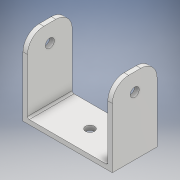
# Autodesk Inventor part: ShoulderPart2
Saved by Autodesk Inventor 2018 (Build 220112000, 112)
## iProperties
Created: 2018-02-09
Part Number: ShoulderPart2
Material: Plastique ABS
Document SubType Name: Modeling
Designer: Thomas
Density: 1.06 g/cm^3
Appearance: Lisse - Blanc
Author: Thomas
Autodesk Inventor part; units mm, degrees
ref_plane "YZ Plane" through (0, 0, 0) normal (1, 0, 0) x (0, 1, 0)
ref_plane "XZ Plane" through (0, 0, 0) normal (0, 1, 0) x (-1, 0, 0)
ref_plane "XY Plane" through (0, 0, 0) normal (0, 0, 1) x (1, 0, 0)
sketch "Esquisse1" plane through (0, 0, 0) normal (0, 0, 1) x (1, 0, 0)
  line L0 (0, 0) -> (98.8, 0)
  line L1 (98.8, 0) -> (98.8, 49.4)
  line L2 (98.8, 49.4) -> (0, 49.4)
  line L3 (0, 49.4) -> (0, 0)
  dimension "d0" = 98.8
  dimension "d1" = 49.4
  constraints: 8 end point, 2 parallel, 1 horizontal, 1 perpendicular
  measures "d0" distance of L1.end L2.end
  measures "d1" distance of L2.end L0.start
extrude "Extrusion1" add sketch "Esquisse1" along normal blind 5
sketch "Esquisse2" plane through (98.8, 0, 0) normal (1, 0, 0) x (0, 0, -1)
  line L0 (0, 49.4) -> (-5, 49.4) projected
  line L1 (-5, 49.4) -> (-66.3, 49.4)
  line L2 (-84.3, 31.4) -> (-84.3, 18)
  line L3 (-66.3, 0) -> (-5, 0)
  line L4 (-5, 0) -> (-5, 49.4)
  arc A0 (-66.3, 49.4) -> (-84.3, 31.4) centre (-66.3, 31.4) ccw
  arc A1 (-84.3, 18) -> (-66.3, 0) centre (-66.3, 18) ccw
  point P0 (0, 0)
  point P1 (-84.3, 49.4)
  dimension "d4" = 79.3
  dimension "d5" = 49.4
  dimension "d6" = 18
  dimension "d7" = 18
  constraints: 8 end point, 4 point on circle, 4 tangent, 2 centre point, 2 parallel, 2 point on line, 1 horizontal, 1 perpendicular
  measures "d4" distance of L0.end point (-84.3, 49.4)
  measures "d5" distance of L3.end L0.end
  measures "d6" radius of A0
  measures "d7" radius of A1
extrude "Extrusion2" add sketch "Esquisse2" against normal blind 5
sketch "Esquisse3" plane through (0, 0, 0) normal (-1, 0, 0) x (0, 0, 1)
  line L0 (66.3, 49.4) -> (5, 49.4) projected
  line L1 (5, 49.4) -> (66.3, 49.4)
  line L2 (84.3, 31.4) -> (84.3, 18)
  line L3 (66.3, 0) -> (5, 0)
  line L4 (5, 0) -> (5, 49.4)
  arc A0 (66.3, 0) -> (84.3, 18) centre (66.3, 18) ccw
  arc A1 (84.3, 31.4) -> (66.3, 49.4) centre (66.3, 31.4) ccw
  point P0 (0, 0)
  point P1 (84.3, 0)
  dimension "d13" = 79.3
  dimension "d14" = 49.4
  dimension "d15" = 18
  constraints: 8 end point, 4 point on circle, 4 tangent, 2 centre point, 2 parallel, 2 point on line, 1 equal radius, 1 horizontal, 1 perpendicular
  measures "d13" distance of point (84.3, 0) L3.end
  measures "d14" distance of L3.end L0.end
  measures "d15" radius of A0
extrude "Extrusion3" add sketch "Esquisse3" against normal blind 5
sketch "Esquisse4" plane through (0, 0, 0) normal (-1, 0, 0) x (0, 0, 1)
  circle A0 centre (64.8, 24.7) radius 5
  line L0 (84.3, 31.4) -> (84.3, 18) projected
  line L1 (0, 0) -> (66.3, 0) projected
  dimension "d18" = 10
  dimension "d19" = 19.5
  dimension "d20" = 24.7
  constraints: 1 centre point
  measures "d18" diameter of A0
  measures "d19" distance from line of L0 A0.centre
  measures "d20" distance from line of L1 A0.centre
extrude "Extrusion4" cut sketch "Esquisse4" against normal blind 5
sketch "Esquisse5" plane through (98.8, 0, 0) normal (1, 0, 0) x (0, 0, -1)
  circle A0 centre (-64.8, 24.7) radius 5
  line L0 (0, 49.4) -> (-66.3, 49.4) projected
  line L1 (-84.3, 31.4) -> (-84.3, 18) projected
  point P0 (0, 0)
  dimension "d23" = 10
  dimension "d24" = 24.7
  dimension "d25" = 19.5
  constraints: 1 centre point
  measures "d23" diameter of A0
  measures "d24" distance from line of L0 A0.centre
  measures "d25" distance from line of L1 A0.centre
extrude "Extrusion5" cut sketch "Esquisse5" against normal blind 5
sketch "Esquisse6" plane through (0, 0, 0) normal (0, 0, -1) x (-1, 0, 0)
  line L0 (-98.8, 49.4) -> (0, 49.4) projected
  line L1 (0, 0) -> (-98.8, 49.4)
  line L2 (-98.8, 0) -> (-98.8, 49.4) projected
  line L3 (-98.8, 0) -> (0, 49.4)
  circle A0 centre (-49.4, 24.7) radius 5
  dimension "d28" = 10
  constraints: 4 end point, 1 centre point, 1 midpoint
  measures "d28" diameter of A0
extrude "Extrusion6" cut sketch "Esquisse6" against normal blind 5 contours A0 L3 L1 | L1 L3 A0 | A0 L1 L3 | L1 A0 L3
fillet "Congé1" radius 2 2 edges at (93.8, 24.7, 5) (5, 24.7, 5)
